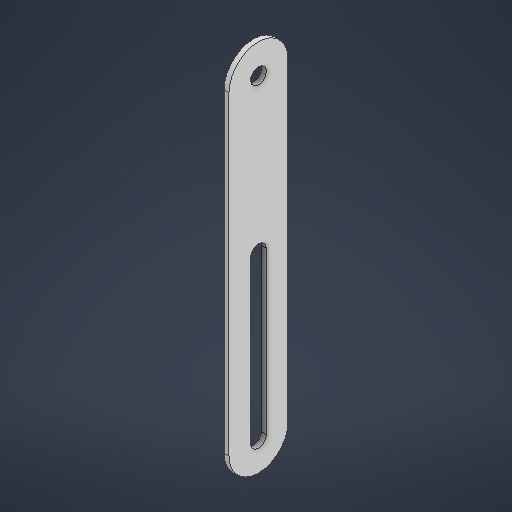
# Autodesk Inventor part: hgsupport
Saved by Autodesk Inventor 2025.2 (Build 292293000, 293)
## iProperties
Created: 2025-04-18
Part Number: hgsupport
Material: Generic
Document SubType Name: Modeling
Designer: roejo
Density: 1 g/cm^3
Appearance: Default
Author: roejo
Autodesk Inventor part; units mm, degrees
ref_plane "YZ Plane" through (0, 0, 0) normal (1, 0, 0) x (0, 1, 0)
ref_plane "XZ Plane" through (0, 0, 0) normal (0, 1, 0) x (-1, 0, 0)
ref_plane "XY Plane" through (0, 0, 0) normal (0, 0, 1) x (1, 0, 0)
sketch "Sketch1" plane through (0, 0, 0) normal (1, 0, 0) x (0, 1, 0)
  circle A0 centre (0, 0) radius 2.54
  arc A1 (0, -9.525) -> (0, 9.525) centre (0, 0) ccw
  line L0 (0, 9.525) -> (-101.6, 9.525)
  line L1 (-101.6, -9.525) -> (0, -9.525)
  arc A2 (-49.53, -2.54) -> (-49.53, 2.54) centre (-49.53, 0) ccw
  line L2 (-49.53, 2.54) -> (-101.6, 2.54)
  line L3 (-49.53, -2.54) -> (-101.6, -2.54)
  arc A3 (-101.6, 2.54) -> (-101.6, -2.54) centre (-101.6, 0) ccw
  arc A4 (-101.6, 9.525) -> (-101.6, -9.525) centre (-101.6, 0) ccw
  point P0 (-111.76, 0)
  dimension "d0" = 5.08
  dimension "d12" = 5.08
  dimension "d17" = 52.07
  constraints: 8 end point, 8 point on circle, 5 centre point, 3 coincident, 3 horizontal, 2 tangent
  measures "d0" diameter of A0
  measures "d12" diameter of A2
  measures "d17" distance of L2.start L2.end
extrude "Extrusion1" add sketch "Sketch1" along normal blind 1.5875
body "Solid1"
